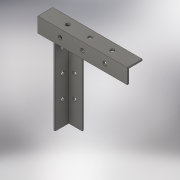
# Autodesk Inventor part: lol
Saved by Autodesk Inventor 2019 (Build 230136000, 136)
## iProperties
Created: 2020-11-14
Part Number: lol
Material: Generic
Document SubType Name: Modeling
Designer: Manoj
Density: 1 g/cm^3
Appearance: Galvanized
Author: Manoj
Autodesk Inventor part; units mm, degrees
ref_plane "YZ Plane" through (0, 0, 0) normal (1, 0, 0) x (0, 1, 0)
ref_plane "XZ Plane" through (0, 0, 0) normal (0, 1, 0) x (-1, 0, 0)
ref_plane "XY Plane" through (0, 0, 0) normal (0, 0, 1) x (1, 0, 0)
sketch "Sketch1" plane through (0, 0, 0) normal (1, 0, 0) x (0, 1, 0)
  line L0 (0, 0) -> (-20, 0)
  line L1 (-20, 0) -> (-20, -2)
  line L2 (-20, -2) -> (0, -2)
  line L3 (0, -2) -> (0, 0)
  line L4 (0, 0) -> (-2, 0)
  line L5 (-2, 0) -> (-2, -20)
  line L6 (-2, -20) -> (0, -20)
  line L7 (0, -20) -> (0, 0)
  dimension "d0" = 20
  dimension "d1" = 2
  dimension "d2" = 2
  dimension "d3" = 20
  constraints: 16 end point, 4 parallel, 2 horizontal, 2 perpendicular
  measures "d0" distance of L2.end L1.end
  measures "d1" distance of L1.end L0.end
  measures "d2" distance of L6.end L5.end
  measures "d3" distance of L5.end L4.end
extrude "Extrusion1" add sketch "Sketch1" along normal blind 120
sketch "Sketch2" plane through (0, 0, 0) normal (0, 1, 0) x (1, 0, 0)
  line L0 (0, 20) -> (0, 0) projected
  line L1 (0, 0) -> (0, 10)
  line L2 (0, 10) -> (30, 10)
  circle A0 centre (30, 10) radius 2.5
  dimension "d6" = 10
  dimension "d7" = 30
  dimension "d8" = 5
  constraints: 4 end point, 1 centre point, 1 coincident, 1 horizontal, 1 midpoint
  measures "d6" distance of L0.end L1.end
  measures "d7" distance of L1.end L2.end
  measures "d8" diameter of A0
extrude "Extrusion2" cut sketch "Sketch2" against normal blind 120
pattern_linear "Rectangular Pattern1" count 3 spacing 30 along (1, 0, 0) of "Extrusion2"
sketch "Sketch3" plane through (0, -20, 0) normal (0, 0, 1) x (1, 0, 0)
  line L0 (0, 0) -> (0, 18) projected
  line L1 (0, 0) -> (0, 10)
  line L2 (0, 10) -> (30, 10)
  circle A0 centre (30, 10) radius 2.5
  point P0 (0, 20)
  dimension "d14" = 10
  dimension "d15" = 30
  dimension "d16" = 5
  constraints: 4 end point, 1 centre point, 1 coincident, 1 perpendicular, 1 point on line
  measures "d14" distance of L0.start L1.end
  measures "d15" distance of L1.end L2.end
  measures "d16" diameter of A0
extrude "Extrusion3" cut sketch "Sketch3" against normal blind 120
pattern_linear "Rectangular Pattern2" count 3 spacing 30 along (1, 0, 0) of "Extrusion3"
sketch "Sketch4" plane through (0, -2, -20) normal (0, -1, 0) x (1, 0, 0)
  line L0 (0, 0) -> (120, 0) projected
  line L1 (21.4627, 0) -> (41.4627, 0)
  line L2 (41.4627, 0) -> (41.4627, 2)
  line L3 (41.4627, 2) -> (21.4627, 2)
  line L4 (21.4627, 2) -> (21.4627, 0)
  line L5 (21.4627, 0) -> (23.4627, 0)
  line L6 (23.4627, 0) -> (23.4627, 20)
  line L7 (23.4627, 20) -> (21.4627, 20)
  line L8 (21.4627, 20) -> (21.4627, 0)
  point P0 (0, 20)
  dimension "d22" = 20
  dimension "d23" = 2
  dimension "d24" = 2
  constraints: 16 end point, 4 parallel, 2 horizontal, 2 perpendicular, 1 point on line
  measures "d22" distance of L3.end L2.end
  measures "d23" distance of L2.end L1.end
  measures "d24" distance of L7.end L6.end
extrude "Extrusion4" add sketch "Sketch4" along normal blind 120
sketch "Sketch5" plane through (23.4627, -2, -2) normal (1, 0, 0) x (0, 0, -1)
  line L0 (0, -18) -> (0, 0) projected
  line L1 (-2, -18) -> (0, -18) projected
  line L2 (-2, -18) -> (-2, -120) projected
  line L3 (16, -120) -> (-2, -120) projected
  line L4 (16, -120) -> (16, 0) projected
  line L5 (0, 0) -> (16, 0) projected
  line L6 (-2, 2) -> (-2, -18) projected
  line L7 (-2, -18) -> (0, -18) projected
  line L8 (0, -18) -> (0, 0) projected
  line L9 (0, 0) -> (18, 0) projected
  line L10 (18, 0) -> (18, 2) projected
  line L11 (18, 2) -> (-2, 2) projected
  line L12 (18, 2) -> (-2, 2) projected
  line L13 (-2, 2) -> (8, 2)
  line L14 (8, 2) -> (8, -28)
  circle A0 centre (8, -28) radius 2.5
  dimension "d27" = 30
  dimension "d28" = 5
  constraints: 4 end point, 1 centre point, 1 coincident, 1 midpoint, 1 perpendicular
  measures "d27" distance of L13.end L14.end
  measures "d28" diameter of A0
extrude "Extrusion5" cut sketch "Sketch5" against normal blind 120 contours A0
pattern_linear "Rectangular Pattern3" count 3 spacing 30 along (0, -1, 0) of "Extrusion5"
sketch "Sketch6" plane through (120, 0, -20) normal (0, 0, -1) x (-1, 0, 0)
  line L0 (98.5373, -2) -> (98.5373, -122) projected
  line L1 (98.5373, -2) -> (98.5373, 0)
  line L2 (98.5373, 0) -> (88.5373, 0)
  line L3 (120, 0) -> (0, 0) projected
  line L4 (88.5373, 0) -> (88.5373, -30)
  circle A0 centre (88.5373, -30) radius 2.5
  dimension "d34" = 10
  dimension "d35" = 30
  dimension "d36" = 5
  constraints: 6 end point, 1 centre point, 1 coincident, 1 perpendicular, 1 point on line, 1 vertical
  measures "d34" distance of L1.end L2.end
  measures "d35" distance of L2.end L4.end
  measures "d36" diameter of A0
extrude "Extrusion6" cut sketch "Sketch6" against normal blind 120
pattern_linear "Rectangular Pattern4" count 3 spacing 30 along (0, -1, 0) of "Extrusion6"
fillet "Fillet1" radius 2 2 edges at (21.4627, -11, -2) (21.4627, -2, -11)
fillet "Fillet2" radius 2 2 edges at (23.4627, -2, -10) (23.4627, -11, -2)
body "Solid1"
